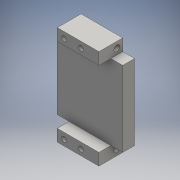
# Autodesk Inventor part: frameBack
Saved by Autodesk Inventor 2016 (Build 200138000, 138)
## iProperties
Created: 2016-05-21
Part Number: frameBack
Material: Generic
Document SubType Name: Modeling
Designer: Henrik Samuelsson
Density: 1 g/cm^3
Appearance: Default
Author: Henrik Samuelsson
Autodesk Inventor part; units mm, degrees
ref_plane "YZ Plane" through (0, 0, 0) normal (1, 0, 0) x (0, 1, 0)
ref_plane "XZ Plane" through (0, 0, 0) normal (0, 1, 0) x (-1, 0, 0)
ref_plane "XY Plane" through (0, 0, 0) normal (0, 0, 1) x (1, 0, 0)
sketch "Sketch1" plane through (0, 0, 0) normal (0, 1, 0) x (-1, 0, 0)
  line L0 (0, 0) -> (66, 0)
  line L1 (66, 0) -> (66, -100)
  line L2 (66, -100) -> (0, -100)
  line L3 (0, -100) -> (0, 0)
  line L4 (66, 0) -> (54, 0)
  line L5 (54, 0) -> (54, -12)
  line L6 (54, -12) -> (66, -12)
  line L7 (66, -12) -> (66, 0)
  line L8 (0, 0) -> (12, 0)
  line L9 (12, 0) -> (12, -12)
  line L10 (12, -12) -> (0, -12)
  line L11 (0, -12) -> (0, 0)
  line L12 (0, -100) -> (12, -100)
  line L13 (12, -100) -> (12, -88)
  line L14 (12, -88) -> (0, -88)
  line L15 (0, -88) -> (0, -100)
  line L16 (66, -100) -> (54, -100)
  line L17 (54, -100) -> (54, -88)
  line L18 (54, -88) -> (66, -88)
  line L19 (66, -88) -> (66, -100)
  dimension "d0" = 66
  dimension "d1" = 100
  dimension "d2" = 12
  dimension "d3" = 12
  dimension "d4" = 12
  dimension "d5" = 12
  dimension "d6" = 12
  dimension "d7" = 12
  dimension "d8" = 12
  dimension "d9" = 12
  constraints: 40 end point, 10 parallel, 5 horizontal, 5 perpendicular
  measures "d0" distance of L1.end L2.end
  measures "d1" distance of L0.end L1.end
  measures "d2" distance of L6.end L5.end
  measures "d3" distance of L5.end L4.end
  measures "d4" distance of L9.end L10.end
  measures "d5" distance of L8.end L9.end
  measures "d6" distance of L14.end L13.end
  measures "d7" distance of L13.end L12.end
  measures "d8" distance of L17.end L18.end
  measures "d9" distance of L16.end L17.end
extrude "Extrusion1" add sketch "Sketch1" along normal blind 12 contours L0 L5 L6 L1 L18 L17 L2 L13 L14 L3 L10 L9
sketch "Sketch2" plane through (-54, 0, 0) normal (-1, 0, 0) x (0, 0, 1)
  circle A0 centre (-6, 6) radius 3
  line L0 (0, 0) -> (-12, 0) projected
  line L1 (0, 12) -> (0, 0) projected
  circle A1 centre (-94, 6) radius 3
  line L2 (-100, 12) -> (-88, 12) projected
  line L3 (-100, 0) -> (-100, 12) projected
  dimension "d12" = 6
  dimension "d13" = 6
  dimension "d14" = 6
  dimension "d15" = 6
  dimension "d16" = 6
  dimension "d17" = 6
  constraints: 2 centre point
  measures "d12" diameter of A0
  measures "d13" distance from line of L0 A0.centre
  measures "d14" distance from line of L1 A0.centre
  measures "d15" diameter of A1
  measures "d16" distance from line of L2 A1.centre
  measures "d17" distance from line of L3 A1.centre
extrude "Extrusion2" cut sketch "Sketch2" against normal up to next
sketch "Sketch3" plane through (0, 0, 0) normal (0, -1, 0) x (1, 0, 0)
  line L0 (-12, 0) -> (-54, 0)
  line L1 (-54, 0) -> (-54, -12)
  line L2 (-54, -12) -> (-12, -12)
  line L3 (-12, -12) -> (-12, 0)
  line L4 (-12, -100) -> (-54, -100) projected
  line L5 (-12, -88) -> (-54, -88)
  line L6 (-54, -88) -> (-54, -100)
  line L7 (-54, -100) -> (-12, -100)
  line L8 (-12, -100) -> (-12, -88)
  point P0 (0, 0)
  constraints: 16 end point, 4 parallel, 2 horizontal, 2 perpendicular
extrude "Extrusion3" add sketch "Sketch3" along normal blind 12
sketch "Sketch4" plane through (0, -12, 0) normal (0, -1, 0) x (1, 0, 0)
  circle A0 centre (-30, -6) radius 2.5
  circle A1 centre (-30, -94) radius 2.5
  circle A2 centre (-47, -94) radius 2.5
  circle A3 centre (-47, -6) radius 2.5
  line L0 (-12, 0) -> (-54, 0) projected
  line L1 (-54, -100) -> (-12, -100) projected
  line L2 (-12, -100) -> (-12, -88) projected
  line L3 (-54, -88) -> (-54, -100) projected
  line L4 (-54, 0) -> (-54, -12) projected
  line L5 (-12, -12) -> (-12, 0) projected
  point P0 (0, 0)
  dimension "d22" = 5
  dimension "d23" = 5
  dimension "d24" = 5
  dimension "d25" = 5
  dimension "d26" = 6
  dimension "d27" = 6
  dimension "d28" = 6
  dimension "d29" = 6
  dimension "d31" = 7
  dimension "d32" = 7
  dimension "d36" = 17
  dimension "d37" = 17
  constraints: 4 centre point
  measures "d22" diameter of A0
  measures "d23" diameter of A1
  measures "d24" diameter of A2
  measures "d25" diameter of A3
  measures "d26" distance from line of L0 A0.centre
  measures "d27" distance from line of L0 A3.centre
  measures "d28" distance from line of A2.centre L1
  measures "d29" distance from line of L1 A1.centre
  measures "d31" distance from line of L3 A2.centre
  measures "d32" distance from line of L4 A3.centre
  measures "d36" distance of A3.centre A0.centre
  measures "d37" distance of A2.centre A1.centre
extrude "Extrusion4" cut sketch "Sketch4" against normal blind 6
body "Solid1"
